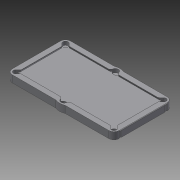
# Autodesk Inventor part: Table_Model
Saved by Autodesk Inventor 2015 (Build 190159000, 159)
## iProperties
Created: 2016-11-24
Part Number: Table_Model
Material: Generic
Document SubType Name: Modeling
Designer: Guy
Density: 1 g/cm^3
Appearance: Default
Author: Guy
Autodesk Inventor part; units mm, degrees
sketch "Sketch1" plane through (0, 0, 0) normal (0, 0, 1) x (1, 0, 0)
  line L0 (0, 0) -> (2051, 0)
  line L1 (2051, 0) -> (2051, 1120.8)
  line L2 (2051, 1120.8) -> (0, 1120.8)
  line L3 (0, 1120.8) -> (0, 0)
  dimension "d0" = 2051
  dimension "d1" = 1120.8
  constraints: 8 end point, 2 parallel, 1 horizontal, 1 perpendicular
  measures "d0" distance of L2.end L1.end
  measures "d1" distance of L2.end L0.start
extrude "Extrusion1" add sketch "Sketch1" along normal blind 134.9
sketch "Sketch2" plane through (0, 0, 134.9) normal (0, 0, 1) x (1, 0, 0)
  line L0 (0, 0) -> (2051, 0) projected
  line L1 (2051, 0) -> (2051, 1120.8) projected
  line L2 (2051, 1120.8) -> (0, 1120.8) projected
  line L3 (0, 1120.8) -> (0, 0) projected
  line L4 (101.6, 100) -> (1949.4, 100)
  line L5 (1949.4, 100) -> (1949.4, 1020.8)
  line L6 (1949.4, 1020.8) -> (101.6, 1020.8)
  line L7 (101.6, 1020.8) -> (101.6, 100)
  dimension "d4" = 1847.8
  dimension "d5" = 920.8
  dimension "d6" = 101.6
  dimension "d7" = 100
  constraints: 8 end point, 2 parallel, 1 horizontal, 1 perpendicular
  measures "d4" distance of L5.end L6.end
  measures "d5" distance of L6.end L4.start
  measures "d6" distance between parallel lines of L3 L7
  measures "d7" distance between parallel lines of L0 L4
extrude "Extrusion2" cut sketch "Sketch2" against normal blind 39.7 contours L7 L6 L5 L4
ref_plane "Work Plane1" through (1025.5, 0, 0) normal (1, 0, 0) x (0, 0, -1)
sketch "Sketch4" plane through (1025.5, 0, 0) normal (1, 0, 0) x (0, 0, -1)
  line L0 (0, 1120.8) -> (0, 0) projected
  line L1 (0, 0) -> (-134.9, 0) projected
  line L2 (-134.9, 1120.8) -> (-134.9, 0) projected
  line L3 (0, 1120.8) -> (-134.9, 1120.8) projected
  line L4 (-134.9, 100) -> (-134.9, 1020.8) projected
  line L5 (-134.9, 100) -> (-134.9, 1020.8) projected
  line L6 (-134.9, 100) -> (-95.2, 100) projected
  line L7 (-95.2, 100) -> (-95.2, 1020.8) projected
  line L8 (-134.9, 1020.8) -> (-95.2, 1020.8) projected
  line L9 (-95.2, 100) -> (-95.2, 87.3)
  line L10 (-95.2, 87.3) -> (-126.96, 100)
  line L11 (-95.2, 1020.8) -> (-95.2, 1033.5)
  line L12 (-95.2, 1033.5) -> (-126.96, 1020.8)
  line L13 (-95.2, 1020.8) -> (-126.96, 1020.8)
  line L14 (-134.9, 1020.8) -> (-95.2, 1020.8) projected
  line L15 (-126.96, 100) -> (-95.2, 100)
  dimension "d20" = 12.7
  dimension "d21" = 7.94
  dimension "d22" = 12.7
  dimension "d23" = 7.94
  constraints: 12 end point, 3 point on line, 1 collinear, 1 horizontal, 1 vertical
  measures "d20" distance of L7.end L11.end
  measures "d21" distance from line of L12.end L2
  measures "d22" distance of L6.end L9.end
  measures "d23" distance of L4.start L10.end
extrude "Extrusion4" cut sketch "Sketch4" along normal mid plane 1848 contours L12 L11 L8 | L6 L9 L10
ref_plane "Work Plane2" through (0, 560.4, 0) normal (0, -1, 0) x (1, 0, 0)
sketch "Sketch6" plane through (0, 560.4, 0) normal (0, -1, 0) x (1, 0, 0)
  line L0 (2051, 0) -> (0, 0) projected
  line L1 (0, 0) -> (0, 134.9) projected
  line L2 (2051, 134.9) -> (0, 134.9) projected
  line L3 (2051, 0) -> (2051, 134.9) projected
  line L4 (101.6, 126.96) -> (101.6, 95.2) projected
  line L5 (101.6, 134.9) -> (101.6, 126.96) projected
  line L6 (1949.4, 134.9) -> (1949.4, 126.96) projected
  line L7 (1949.4, 126.96) -> (1949.4, 95.2) projected
  line L8 (1949.4, 95.2) -> (1962.1, 95.2)
  line L9 (1962.1, 95.2) -> (1949.4, 126.96)
  line L10 (1949.4, 126.96) -> (1949.4, 95.2)
  line L11 (101.6, 95.2) -> (88.9, 95.2)
  line L12 (88.9, 95.2) -> (101.6, 126.96)
  line L13 (101.6, 95.2) -> (101.6, 126.96)
  point P0 (0, 0)
  dimension "d39" = 12.7
  dimension "d40" = 12.7
  constraints: 12 end point, 2 collinear, 2 horizontal
  measures "d39" distance of L7.end L8.end
  measures "d40" distance of L4.end L11.end
extrude "Extrusion6" cut sketch "Sketch6" along normal mid plane 921 contours L4 L11 L12 | L9 L8 L7
sketch "Sketch7" plane through (0, 0, 134.9) normal (0, 0, 1) x (1, 0, 0)
  arc A0 (107.161, 1120.5433) -> (0.2098, 1014.3264) centre (100, 1020.8) ccw
  line L0 (0, 1120.8) -> (0, 0) projected
  line L1 (2051, 1120.8) -> (0, 1120.8) projected
  circle A1 centre (84.3045, 1036.5) radius 49.2
  line L2 (49.5197, 1071.2946) -> (29.2994, 1091.5207)
  line L3 (0, 1120.8) -> (0, 0) projected
  line L4 (0, 1020.8) -> (0, 1120.8)
  line L5 (0, 1120.8) -> (100, 1120.8)
  line L6 (1025.5, 1317.5448) -> (1025.5, -400.2984)
  line L7 (2051, 0) -> (2051, 1120.8) projected
  line L8 (2051, 1120.8) -> (2051, 0)
  line L9 (0, 1120.8) -> (2051, 1120.8)
  line L10 (-695.8087, 560.4) -> (2268.6576, 560.4)
  line L11 (0, 0) -> (2051, 0) projected
  line L12 (0, 0) -> (0, 1120.8)
  circle A2 centre (1966.7, 84.3045) radius 49.2
  arc A3 (1943.839, 0.2567) -> (2050.7902, 106.4736) centre (1951, 100) ccw
  line L13 (0, 0) -> (2051, 0)
  arc A4 (2051, 1020.8) -> (1951, 1120.8) centre (1951, 1020.8) ccw
  circle A5 centre (1966.7, 1036.4955) radius 49.2
  line L14 (2001.4946, 1071.2803) -> (2021.7207, 1091.5006)
  line L15 (2051, 1120.8) -> (1951, 1120.8)
  line L16 (2051, 1120.8) -> (0, 1120.8) projected
  line L17 (2051, 1120.8) -> (2051, 1020.8)
  line L18 (2051, 0) -> (2051, 1120.8) projected
  arc A6 (0, 100) -> (100, 0) centre (100, 100) ccw
  circle A7 centre (84.3, 84.3045) radius 49.2
  line L19 (49.5054, 49.5197) -> (29.2793, 29.2994)
  line L20 (0, 0) -> (100, 0)
  line L21 (0, 0) -> (0, 100)
  line L22 (2021.7207, 29.2994) -> (2001.4946, 49.5197)
  line L23 (2051, 0) -> (2051, 100)
  line L24 (2051, 0) -> (1951, 0)
  dimension "d45" = 98.4
  dimension "d63" = 98.4
  dimension "d64" = 98.4
  dimension "d68" = 98.4
  dimension "d43" = 100
  dimension "d44" = 28.6
  dimension "d46" = 84.3
  dimension "d47" = 84.3045
  dimension "d58" = 1025.5
  dimension "d59" = 560.4
  dimension "d60" = 100
  dimension "d61" = 28.6
  dimension "d62" = 84.3
  dimension "d65" = 28.6
  dimension "d66" = 84.3
  dimension "d67" = 100
  dimension "d69" = 28.6
  dimension "d70" = 100
  dimension "d71" = 84.3
  constraints: 36 end point, 18 point on circle, 9 point on line, 9 tangent, 6 symmetric about line, 4 centre point, 4 line through centre, 2 collinear, 2 parallel, 1 horizontal, 16 other
  measures "d43" radius of A0
  measures "d44" distance of L2.start L2.end
  measures "d46" distance from line of L1 point (84.304, 1036.5)
  measures "d47" distance from line of L0 point (84.304, 1036.5)
  measures "d58" distance between parallel lines of L6 L7
  measures "d59" distance between parallel lines of L11 L10
  measures "d60" radius of A4
  measures "d61" distance of L14.start L14.end
  measures "d62" distance from line of L7 point (1966.7, 1036.496)
  measures "d65" distance of L19.start L19.end
  measures "d66" distance from line of L0 point (84.3, 84.304)
  measures "d67" radius of A6
  measures "d69" distance of L22.start L22.end
  measures "d70" radius of A3
  measures "d71" distance from line of L8 point (1966.7, 84.304)
extrude "Extrusion7" cut sketch "Sketch7" against normal through all contours A0 L0 L1 | L1 L7 A4 | A6 L11 L0 | A3 L7 L11
extrude "Extrusion8" cut sketch "Sketch7" against normal blind 70 contours A1 | A2 | A5 | A7
sketch "Sketch8" plane through (0, 0, 134.9) normal (0, 0, 1) x (1, 0, 0)
  arc A0 (130.9322, 1020.8) -> (101.6, 990.4402) centre (84.3045, 1036.5) ccw projected
  line L0 (130.9322, 1020.8) -> (1920.0707, 1020.8) projected
  line L1 (1949.4, 990.4374) -> (1949.4, 130.3626) projected
  line L2 (1920.0707, 100) -> (130.9293, 100) projected
  line L3 (101.6, 130.3626) -> (101.6, 990.4402) projected
  arc A1 (100, 1120.8) -> (0, 1020.8) centre (100, 1020.8) ccw projected
  line L4 (0, 1020.8) -> (0, 100) projected
  line L5 (100, 0) -> (1951, 0) projected
  line L6 (2051, 100) -> (2051, 1020.8) projected
  line L7 (1951, 1120.8) -> (100, 1120.8) projected
  circle A2 centre (84.3045, 1036.5) radius 49.2 projected
  line L8 (118.7702, 1071.6106) -> (170.5314, 1020.8)
  arc A3 (130.9322, 1020.8) -> (101.6, 990.4402) centre (84.3045, 1036.5) ccw projected
  line L9 (130.9322, 1020.8) -> (170.5314, 1020.8)
  line L10 (130.9322, 1020.8) -> (1949.4, 1020.8) projected
  line L11 (101.6, 950.5788) -> (101.6, 990.4402)
  line L12 (101.6, 950.5788) -> (49.8387, 1001.3894)
  arc A4 (2051, 1020.8) -> (1951, 1120.8) centre (1951, 1020.8) ccw projected
  arc A5 (0, 100) -> (100, 0) centre (100, 100) ccw projected
  arc A6 (1951, 0) -> (2051, 100) centre (1951, 100) ccw projected
  arc A7 (1949.4, 990.4374) -> (1920.0707, 1020.8) centre (1966.7, 1036.4955) ccw projected
  arc A8 (1920.0707, 100) -> (1949.4, 130.3626) centre (1966.7, 84.3045) ccw projected
  arc A9 (101.6, 130.3626) -> (130.9293, 100) centre (84.3, 84.3045) ccw projected
  line L13 (1932.2361, 1071.6079) -> (1880.4722, 1020.8)
  line L14 (1920.0707, 1020.8) -> (1880.4722, 1020.8)
  arc A10 (1949.4, 990.4374) -> (1920.0707, 1020.8) centre (1966.7, 1036.4955) ccw projected
  line L15 (2001.1639, 1001.3832) -> (1949.4, 950.5753)
  line L16 (1949.4, 950.5753) -> (1949.4, 990.4374)
  line L17 (1949.4, 170.2247) -> (2001.1639, 119.4168)
  arc A11 (1920.0707, 100) -> (1949.4, 130.3626) centre (1966.7, 84.3045) ccw projected
  line L18 (1949.4, 170.2247) -> (1949.4, 130.3626)
  line L19 (1920.0707, 100) -> (1880.4722, 100)
  line L20 (1920.0707, 100) -> (130.9293, 100) projected
  line L21 (1880.4722, 100) -> (1932.2361, 49.1921)
  line L22 (101.6, 130.3626) -> (101.6, 170.2248)
  line L23 (101.6, 130.3626) -> (101.6, 990.4402) projected
  line L24 (101.6, 170.2248) -> (49.8361, 119.4168)
  line L25 (130.9293, 100) -> (170.5278, 100)
  line L26 (170.5278, 100) -> (118.7639, 49.1921)
  arc A12 (101.6, 130.3626) -> (130.9293, 100) centre (84.3, 84.3045) ccw projected
  point P0 (0, 0)
  dimension "d57" = 98.4
  dimension "d74" = 98.4
  dimension "d77" = 98.4
  dimension "d78" = 98.4
  constraints: 32 end point, 15 point on circle, 11 tangent, 10 point on line, 4 parallel, 2 collinear, 1 vertical
  measures "d57" distance of L8.end L11.start
  measures "d74" distance of L13.end L15.end
  measures "d77" distance of L17.start L19.end
  measures "d78" distance of L25.end L22.end
extrude "Extrusion9" cut sketch "Sketch8" against normal blind 39.7 contours A0 L8 L0 | L3 L12 A0 | L13 A7 L0 | L3 A9 L24 | L15 L1 A7 | A9 L2 L26 | L17 A8 L1 | L2 A8 L21
sketch "Sketch9" plane through (0, 0, 134.9) normal (0, 0, 1) x (1, 0, 0)
  arc A0 (2051, 1020.8) -> (1951, 1120.8) centre (1951, 1020.8) ccw projected
  line L0 (1951, 1120.8) -> (100, 1120.8) projected
  arc A1 (100, 1120.8) -> (0, 1020.8) centre (100, 1020.8) ccw projected
  line L1 (0, 1020.8) -> (0, 100) projected
  arc A2 (0, 100) -> (100, 0) centre (100, 100) ccw projected
  line L2 (100, 0) -> (1951, 0) projected
  arc A3 (1951, 0) -> (2051, 100) centre (1951, 100) ccw projected
  line L3 (2051, 100) -> (2051, 1020.8) projected
  line L4 (1949.4, 170.2247) -> (2001.1639, 119.4168) projected
  arc A4 (1932.2361, 49.1921) -> (2001.1639, 119.4168) centre (1966.7, 84.3045) ccw projected
  line L5 (1932.2361, 49.1921) -> (1880.4722, 100) projected
  line L6 (1880.4722, 100) -> (170.5278, 100) projected
  line L7 (170.5278, 100) -> (118.7639, 49.1921) projected
  arc A5 (49.8361, 119.4168) -> (118.7639, 49.1921) centre (84.3, 84.3045) ccw projected
  line L8 (49.8361, 119.4168) -> (101.6, 170.2248) projected
  line L9 (101.6, 170.2248) -> (101.6, 950.5788) projected
  line L10 (101.6, 950.5788) -> (49.8387, 1001.3894) projected
  arc A6 (118.7702, 1071.6106) -> (49.8387, 1001.3894) centre (84.3045, 1036.5) ccw projected
  line L11 (118.7702, 1071.6106) -> (170.5314, 1020.8) projected
  line L12 (170.5314, 1020.8) -> (1880.4722, 1020.8) projected
  line L13 (1880.4722, 1020.8) -> (1932.2361, 1071.6079) projected
  arc A7 (2001.1639, 1001.3832) -> (1932.2361, 1071.6079) centre (1966.7, 1036.4955) ccw projected
  line L14 (2001.1639, 1001.3832) -> (1949.4, 950.5753) projected
  line L15 (1949.4, 950.5753) -> (1949.4, 170.2247) projected
  line L16 (170.5314, 1020.8) -> (1880.4722, 1020.8) projected
  line L17 (934.2, 1020.8) -> (1116.8, 1020.8)
  line L18 (965, 1052.5) -> (1086, 1052.5)
  line L19 (965, 1052.5) -> (934.2, 1020.8)
  line L20 (1086, 1052.5) -> (1116.8, 1020.8)
  arc A8 (1116.8, 1120.8) -> (934.2, 1120.8) centre (1025.5, 901.605) ccw
  line L21 (1025.5, 1139.0542) -> (1025.5, 1110.4542)
  line L22 (1116.8, 1020.8) -> (1116.8, 1120.8)
  arc A9 (1086.1664, 1052.3287) -> (964.8336, 1052.3287) centre (1025.5, 1049.7322) ccw
  arc A10 (964.8336, 1052.3287) -> (1086.1664, 1052.3287) centre (1025.5, 1083.2434) ccw
  line L23 (1025.5, 1015.1542) -> (1025.5, 1110.4542)
  line L24 (-206.9931, 560.4) -> (2183.3755, 560.4)
  line L25 (965, 68.3) -> (1086, 68.3)
  line L26 (965, 68.3) -> (934.2, 100)
  line L27 (1086, 68.3) -> (1116.8, 100)
  arc A11 (934.2, 0) -> (1116.8, 0) centre (1025.5, 219.195) ccw
  line L28 (1025.5, -18.2542) -> (1025.5, 10.3458)
  line L29 (1116.8, 100) -> (1116.8, 0)
  arc A12 (964.8336, 68.4713) -> (1086.1664, 68.4713) centre (1025.5, 71.0678) ccw
  arc A13 (1086.1664, 68.4713) -> (964.8336, 68.4713) centre (1025.5, 37.5566) ccw
  line L30 (934.2, 100) -> (1116.8, 100)
  line L31 (1880.4722, 100) -> (170.5278, 100) projected
  line L32 (934.2, 0) -> (1116.8, 0)
  point P0 (0, 0)
  dimension "d81" = 182.6
  dimension "d82" = 121
  dimension "d84" = 31.7
  dimension "d86" = 28.6
  dimension "d92" = 95.3
  dimension "d95" = 560.4
  dimension "d96" = 28.6
  dimension "d97" = 31.7
  constraints: 30 end point, 17 point on circle, 13 symmetric about line, 8 point on line, 6 centre point, 2 collinear, 1 horizontal, 1 line through centre, 1 parallel, 1 perpendicular, 3 other
  measures "d81" distance of L17.start L17.end
  measures "d82" distance of L18.start L18.end
  measures "d84" distance between parallel lines of L17 L18
  measures "d86" distance of L21.start L21.end
  measures "d92" distance of L21.end L23.start
  measures "d95" distance between parallel lines of L2 L24
  measures "d96" distance of L28.start L28.end
  measures "d97" distance between parallel lines of L25 L6
extrude "Extrusion10" add sketch "Sketch9" against normal blind 134.9 contours L0 L21 A8 | L0 A8 L21 | A11 L28 L2 | L28 A11 L2
extrude "Extrusion11" cut sketch "Sketch9" against normal blind 39.7 contours L12 A10 L20 | L12 L23 L18 L20 A10 | A10 L12 L19 | L19 L18 L23 L12 A10 | L27 A13 L6 | A13 L27 L25 L26 L6 | L26 L6 A13
extrude "Extrusion12" cut sketch "Sketch9" against normal blind 70 contours L23 L18 L19 A9 | A9 L20 L18 L23 | A10 L23 L12 | L12 L23 L18 L20 A10 | L19 L18 L23 L12 A10 | L23 A10 L12 | A12 L26 L25 L27 | A13 L27 L25 L26 L6 | L6 A13
sketch "Sketch10" plane through (2051, 100, 0) normal (1, 0, 0) x (0, 0, -1)
  line L0 (0, 920.8) -> (-134.9, 920.8) projected
  line L1 (-134.9, 0) -> (-134.9, 920.8) projected
  line L2 (0, 0) -> (-134.9, 0) projected
  line L3 (0, 0) -> (0, 920.8) projected
  line L4 (-123.8, 43.7) -> (0, 43.7)
  line L5 (0, 43.7) -> (0, 877.1)
  line L6 (0, 877.1) -> (-123.8, 877.1)
  line L7 (-123.8, 877.1) -> (-123.8, 43.7)
  line L8 (0, 0) -> (0, 920.8) projected
  line L9 (-134.9, -118.2542) -> (0, -118.2542) projected
  line L10 (-134.9, 1039.0542) -> (0, 1039.0542) projected
  line L11 (0, -100) -> (-134.9, -100) projected
  line L12 (0, 1020.8) -> (-134.9, 1020.8) projected
  line L13 (-123.8, 43.7) -> (-123.8, 0)
  line L14 (-123.8, 877.1) -> (-123.8, 920.8)
  line L15 (-134.9, 920.8) -> (-123.8, 920.8)
  line L16 (0, 920.8) -> (-134.9, 920.8) projected
  line L17 (-134.9, 920.8) -> (-134.9, 0)
  line L18 (-134.9, 0) -> (-123.8, 0)
  line L19 (-123.8, 0) -> (0, 0)
  line L20 (0, 0) -> (0, 43.7)
  line L21 (0, 43.7) -> (-123.8, 43.7)
  line L22 (-123.8, 43.7) -> (-123.8, 0)
  line L23 (-123.8, 877.1) -> (0, 877.1)
  line L24 (0, 877.1) -> (0, 920.8)
  line L25 (0, 920.8) -> (-123.8, 920.8)
  line L26 (-123.8, 920.8) -> (-123.8, 877.1)
  dimension "d98" = 833.4
  dimension "d101" = 143.7
  dimension "d102" = 11.1
  constraints: 34 end point, 6 parallel, 4 collinear, 3 horizontal, 3 perpendicular, 2 point on line, 2 vertical
  measures "d98" distance of L6.end L4.start
  measures "d101" distance between parallel lines of L11 L4
  measures "d102" distance between parallel lines of L1 L7
extrude "Extrusion13" cut sketch "Sketch10" against normal blind 10 contours L3 L6 L14 L0 | L3 L2 L13 L4
extrude "Extrusion14" add sketch "Sketch10" along normal blind 10 contours L14 L7 L13 L2 L1 L0
ref_plane "Work Plane3" through (2051, 560.4, 134.9) normal (0, 1, 0) x (1, 0, 0)
sketch "Sketch11" plane through (2051, 560.4, 134.9) normal (0, 1, 0) x (1, 0, 0)
  line L0 (0, 11.1) -> (0, 0) projected
  line L1 (0, 11.1) -> (10, 11.1) projected
  line L2 (10, 0) -> (10, 11.1) projected
  line L3 (0, 0) -> (10, 0) projected
  arc A0 (0, 0) -> (10, 11.1) centre (-1.1605, 11.1) ccw
  line L4 (0, 0) -> (0, 11.1)
  line L5 (0, 11.1) -> (10, 11.1)
  line L6 (10, 11.1) -> (0, 11.1)
  point P0 (-2051, 134.9)
  constraints: 6 end point, 2 point on circle, 1 centre point, 1 collinear, 1 perpendicular, 1 tangent, 1 vertical
extrude "Extrusion15" cut sketch "Sketch11" along normal through all both and the other way through all contours A0 L2 L3
body "Solid1"
